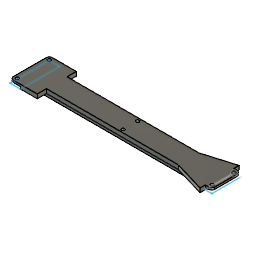
Carsen x10eb Mount1 (Autodesk Fusion 360 design; units mm, degrees)
part number: 2026-08-02-16-37-13-928
Autodesk Fusion 360 part; units mm, degrees
sketch "Skizze1" plane through (0, 0, 0) normal (0, 0, 1) x (1, 0, 0)
  line L0 (0, 27.8) -> (3.3, 27.8)
  line L1 (6.3, 24.8) -> (6.3, 3)
  line L2 (3.3, 0) -> (0, 0)
  line L3 (0, 0) -> (0, 27.8)
  circle A0 centre (3.3, 24.3) radius 1.575
  circle A1 centre (3.3, 3.5) radius 1.575
  line L4 (0, -5.025) -> (-180.6991, -5.025)
  line L5 (-183.6991, -2.025) -> (-183.6991, 29.825)
  line L6 (-180.6991, 32.825) -> (0, 32.825)
  line L7 (0, 32.825) -> (0, -5.025)
  circle A2 centre (-180.1991, 29.325) radius 1.575
  circle A3 centre (-180.1991, -1.525) radius 1.575
  arc A4 (6.3, 24.8) -> (3.3, 27.8) centre (3.3, 24.8) ccw
  arc A5 (3.3, 0) -> (6.3, 3) centre (3.3, 3) ccw
  arc A6 (-180.6991, 32.825) -> (-183.6991, 29.825) centre (-180.6991, 29.825) ccw
  arc A7 (-183.6991, -2.025) -> (-180.6991, -5.025) centre (-180.6991, -2.025) ccw
  line L8 (0, 23.9) -> (-183.6991, 23.9)
  line L9 (-183.6991, 23.9) -> (-183.6991, 3.9)
  line L10 (-183.6991, 3.9) -> (0, 3.9)
  line L11 (0, 3.9) -> (0, 23.9)
  line L12 (0, -5.025) -> (-30, 3.9)
  line L13 (0, 32.825) -> (-30, 23.9)
  line L14 (-30, 23.9) -> (-30, 32.825)
  line L15 (-30, -5.025) -> (-30, 3.9)
  line L16 (-157.4811, -5.025) -> (-157.4811, 3.9)
  line L17 (-157.4811, 23.9) -> (-157.4811, 32.825)
  dimension "d24" = 27.8
  dimension "d25" = 3.15
  dimension "d26" = 3.15
  dimension "d27" = 3.5
  dimension "d28" = 3.5
  dimension "d29" = 3
  dimension "d31" = 6.3
  dimension "d32" = 37.85
  dimension "d38" = 3.15
  dimension "d39" = 3.15
  dimension "d40" = 3.5
  dimension "d41" = 3.5
  dimension "d42" = 3.5
  dimension "d50" = 3
  dimension "d51" = 3
  dimension "d52" = 3
  dimension "d53" = 189.9991
  dimension "d54" = 8.925
  dimension "d55" = 8.925
  dimension "d56" = 30
  dimension "d57" = 30
  constraint horizontal L0
  constraint vertical L1
  constraint horizontal L2
  constraint vertical L3
  constraint vertical A0.centre A1.centre
  constraint horizontal L2.end L3.start
  constraint horizontal L4
  constraint vertical L5
  constraint horizontal L6
  constraint vertical L7
  constraint coincident L3 L4.start
  constraint midpoint L3 L7
  constraint vertical A2.centre A3.centre
  constraint tangent L0 A4
  constraint tangent L1 A4
  constraint tangent L1 A5
  constraint tangent L2 A5
  constraint tangent L6 A6
  constraint tangent L5 A6
  constraint tangent L5 A7
  constraint tangent L4 A7
  constraint equal A6 A7
  constraint vertical L2.end L4.start
  constraint horizontal L8
  constraint vertical L9
  constraint horizontal L10
  constraint vertical L11
  constraint coincident L5 L9.end
  constraint coincident L3 L8.start
  constraint coincident L10 L12.end
  constraint coincident L8 L13.end
  constraint coincident L6 L14.end
  constraint perpendicular L6 L14
  constraint perpendicular L4 L15
  constraint coincident L4 L15.start
  constraint coincident L4 L16.start
  constraint perpendicular L4 L16
  constraint coincident L10 L16.end
  constraint coincident L8 L17.start
  constraint perpendicular L8 L17
  constraint coincident L6 L17.end
  measures "d24" distance of L0 L2
  measures "d25" diameter of A0
  measures "d26" diameter of A1
  measures "d27" distance of L2 A1.centre
  measures "d28" distance of L0 A0.centre
  measures "d29" distance of L1 A0.centre
  measures "d31" distance of L1 L3
  measures "d32" distance of L4 L6
  measures "d38" diameter of A2
  measures "d39" diameter of A3
  measures "d40" distance of L6 A2.centre
  measures "d41" distance of L4 A3.centre
  measures "d42" distance of L5 A2.centre
  measures "d50" radius of A4
  measures "d51" radius of A5
  measures "d52" radius of A6
  measures "d53" distance of L1 L5
  measures "d54" distance of L4 L10
  measures "d55" distance of L6 L8
  measures "d56" horizontal distance of L4.start L12.end
  measures "d57" horizontal distance of L6.end L13.end
extrude "Extrusion8" add sketch "Skizze1" along normal blind 4 contours L0 L1 L2 L3 L7 A4 A5 L11 | L3 L7 L8 L13 | L3 L5 L7 L8 L9 L10 L11 | L3 L7 L10 L12 | L5 L6 A6 L8 L17 | L4 L5 A7 L10 L16
sketch "Skizze4" plane through (0, 0, 4) normal (0, 0, 1) x (-1, 0, 0)
  circle A0 centre (180.1991, 1.525) radius 1.575
  circle A1 centre (180.1991, -29.325) radius 1.575
  circle A2 centre (-3.3, -24.3) radius 1.575
  circle A3 centre (-3.3, -3.5) radius 1.575
  line L0 (0, -32.825) -> (30, -23.9)
  line L1 (30, -23.9) -> (157.4811, -23.9)
  line L2 (157.4811, -23.9) -> (157.4811, -32.825)
  line L3 (157.4811, -32.825) -> (180.6991, -32.825)
  arc A4 (180.6991, -32.825) -> (183.6991, -29.825) centre (180.6991, -29.825) ccw
  line L4 (183.6991, -29.825) -> (183.6991, -23.9)
  line L5 (183.6991, -23.9) -> (183.6991, -3.9)
  line L6 (183.6991, -3.9) -> (183.6991, 2.025)
  arc A5 (183.6991, 2.025) -> (180.6991, 5.025) centre (180.6991, 2.025) ccw
  line L7 (180.6991, 5.025) -> (157.4811, 5.025)
  line L8 (157.4811, 5.025) -> (157.4811, -3.9)
  line L9 (157.4811, -3.9) -> (30, -3.9)
  line L10 (30, -3.9) -> (0, 5.025)
  line L11 (0, 5.025) -> (0, 0)
  line L12 (0, 0) -> (-3.3, 0)
  arc A6 (-3.3, 0) -> (-6.3, -3) centre (-3.3, -3) ccw
  line L13 (-6.3, -3) -> (-6.3, -24.8)
  arc A7 (-6.3, -24.8) -> (-3.3, -27.8) centre (-3.3, -24.8) ccw
  line L14 (-3.3, -27.8) -> (0, -27.8)
  line L15 (0, -27.8) -> (0, -32.825)
  circle A8 centre (86.2, -6.9) radius 1.575
  circle A9 centre (86.2, -20.9) radius 1.575
  dimension "d60" = 3.15
  dimension "d61" = 92.5
  dimension "d63" = 3
  dimension "d64" = 3.15
  dimension "d65" = 92.5
  dimension "d66" = 3
  measures "d60" diameter of A8
  measures "d61" distance of L13 A8.centre
  measures "d63" distance of L9 A8.centre
  measures "d64" diameter of A9
  measures "d65" distance of L13 A9.centre
  measures "d66" distance of L1 A9.centre
extrude "Extrusion9" cut sketch "Skizze4" against normal blind 4 contours A8 | A9
sketch "Skizze5" plane through (0, 0, 0) normal (0, 0, -1) x (1, 0, 0)
  circle A0 centre (-86.2, -6.9) radius 1.575
  circle A1 centre (-86.2, -20.9) radius 1.575
  circle A2 centre (3.3, -3.5) radius 1.575
  circle A3 centre (-180.1991, -29.325) radius 1.575
  circle A4 centre (3.3, -24.3) radius 1.575
  circle A5 centre (-180.1991, 1.525) radius 1.575
  line L0 (-30, -23.9) -> (0, -32.825)
  line L1 (0, -32.825) -> (0, -27.8)
  line L2 (0, -27.8) -> (3.3, -27.8)
  arc A6 (3.3, -27.8) -> (6.3, -24.8) centre (3.3, -24.8) ccw
  line L3 (6.3, -24.8) -> (6.3, -3)
  arc A7 (6.3, -3) -> (3.3, 0) centre (3.3, -3) ccw
  line L4 (3.3, 0) -> (0, 0)
  line L5 (0, 0) -> (0, 5.025)
  line L6 (0, 5.025) -> (-30, -3.9)
  line L7 (-30, -3.9) -> (-157.4811, -3.9)
  line L8 (-157.4811, -3.9) -> (-157.4811, 5.025)
  line L9 (-157.4811, 5.025) -> (-180.6991, 5.025)
  arc A8 (-180.6991, 5.025) -> (-183.6991, 2.025) centre (-180.6991, 2.025) ccw
  line L10 (-183.6991, 2.025) -> (-183.6991, -3.9)
  line L11 (-183.6991, -3.9) -> (-183.6991, -23.9)
  line L12 (-183.6991, -23.9) -> (-183.6991, -29.825)
  arc A9 (-183.6991, -29.825) -> (-180.6991, -32.825) centre (-180.6991, -29.825) ccw
  line L13 (-180.6991, -32.825) -> (-157.4811, -32.825)
  line L14 (-157.4811, -32.825) -> (-157.4811, -23.9)
  line L15 (-157.4811, -23.9) -> (-30, -23.9)
  line L16 (0, -27.8) -> (6.5, -27.8)
  line L17 (6.5, -27.8) -> (6.5, 0)
  line L18 (6.5, 0) -> (0, 0)
  line L19 (0, 0) -> (0, -27.8)
  line L20 (-183.6991, -32.9017) -> (-173.6991, -32.9017)
  line L21 (-173.6991, -32.9017) -> (-173.6991, 5.078)
  line L22 (-173.6991, 5.078) -> (-183.6991, 5.078)
  line L23 (-183.6991, 5.078) -> (-183.6991, -32.9017)
  dimension "d69" = 10
  constraint horizontal L16
  constraint vertical L17
  constraint horizontal L18
  constraint vertical L19
  constraint coincident L1.end L2.start
  constraint horizontal L20
  constraint vertical L21
  constraint horizontal L22
  constraint vertical L23
  measures "d69" distance of L20.start L20.end
extrude "Extrusion10" cut sketch "Skizze5" against normal blind 2 contours L9 A8 L10 L11 L12 A9 L13 L21 L23
extrude "Extrusion11" cut sketch "Skizze5" against normal blind 2 contours L2 A6 L3 A7 L4 L16 L18 L19
sketch "Skizze6" plane through (0, 0, 0) normal (0, 0, -1) x (1, 0, 0)
  line L0 (-1.6975, -23.4) -> (-173.6975, -23.4)
  line L1 (-173.6975, -23.4) -> (-173.6975, -20.4)
  line L2 (-173.6975, -20.4) -> (-1.6975, -20.4)
  line L3 (-1.6975, -20.4) -> (-1.6975, -23.4)
  line L4 (0, 0) -> (0, -27.8)
  line L5 (-173.6991, -32.9017) -> (-173.6991, 5.078)
  line L6 (-157.4811, -23.9) -> (-30, -23.9)
  line L7 (-1.641, -4.4) -> (-173.641, -4.4)
  line L8 (-173.641, -4.4) -> (-173.641, -7.4)
  line L9 (-173.641, -7.4) -> (-1.641, -7.4)
  line L10 (-1.641, -7.4) -> (-1.641, -4.4)
  line L11 (-30, -3.9) -> (-157.4811, -3.9)
  line L12 (-73.2, -20.4) -> (-76.2, -20.4)
  line L13 (-76.2, -20.4) -> (-76.2, -7.4)
  line L14 (-76.2, -7.4) -> (-73.2, -7.4)
  line L15 (-73.2, -7.4) -> (-73.2, -20.4)
  line L16 (-33.3271, -20.4) -> (-73.2, -8.955)
  line L17 (-67.7437, -7.4) -> (-22.4534, -20.4)
  line L18 (-76.2, -20.4) -> (-96.2, -20.4)
  line L19 (-96.2, -20.4) -> (-96.2, -19)
  line L20 (-96.2, -19) -> (-76.2, -19)
  line L21 (-76.2, -19) -> (-76.2, -20.4)
  line L22 (-76.2, -7.4) -> (-96.2, -7.4)
  line L23 (-96.2, -7.4) -> (-96.2, -8.8)
  line L24 (-96.2, -8.8) -> (-76.2, -8.8)
  line L25 (-76.2, -8.8) -> (-76.2, -7.4)
  line L26 (-173.6975, -23.4) -> (-168.6975, -23.4)
  line L27 (-168.6975, -23.4) -> (-168.6975, -7.4)
  line L28 (-168.6975, -7.4) -> (-173.6975, -7.4)
  line L29 (-173.6975, -7.4) -> (-173.6975, -23.4)
  line L30 (-22.4534, -20.4) -> (-27.4534, -20.4)
  line L31 (-27.4534, -20.4) -> (-27.4534, -7.4)
  line L32 (-27.4534, -7.4) -> (-22.4534, -7.4)
  line L33 (-22.4534, -7.4) -> (-22.4534, -20.4)
  line L34 (-168.6975, -20.4) -> (-99.2, -8.9486)
  line L35 (-168.6975, -17.3595) -> (-108.2541, -7.4)
  line L36 (-96.2, -20.4) -> (-99.2, -20.4)
  line L37 (-99.2, -20.4) -> (-99.2, -7.4)
  line L38 (-99.2, -7.4) -> (-96.2, -7.4)
  line L39 (-96.2, -7.4) -> (-96.2, -20.4)
  point P0 (-86.2, -20.9)
  dimension "d74" = 172
  dimension "d75" = 3
  dimension "d76" = 173.6991
  dimension "d78" = 0.5
  dimension "d81" = 3
  dimension "d82" = 0.5
  dimension "d83" = 3
  dimension "d85" = 10
  dimension "d88" = 3
  dimension "d90" = 20
  dimension "d91" = 1.4
  dimension "d92" = 5
  dimension "d93" = 172
  dimension "d96" = 3
  dimension "d101" = 5
  dimension "d102" = 13
  constraint horizontal L0
  constraint vertical L1
  constraint horizontal L2
  constraint vertical L3
  constraint horizontal L7
  constraint vertical L8
  constraint horizontal L9
  constraint vertical L10
  constraint horizontal L12
  constraint vertical L13
  constraint horizontal L14
  constraint vertical L15
  constraint coincident L2 L12.start
  constraint coincident L2 L16.start
  constraint coincident L15 L16.end
  constraint coincident L9 L17.start
  constraint coincident L2 L17.end
  constraint parallel L16 L17
  constraint horizontal L18
  constraint vertical L19
  constraint horizontal L20
  constraint vertical L21
  constraint horizontal L22
  constraint vertical L23
  constraint horizontal L24
  constraint vertical L25
  constraint horizontal L26
  constraint vertical L27
  constraint horizontal L28
  constraint vertical L29
  constraint horizontal L30
  constraint vertical L31
  constraint horizontal L32
  constraint vertical L33
  constraint coincident L9 L31.end
  constraint coincident L27 L34.start
  constraint coincident L2 L34.start
  constraint coincident L27 L35.start
  constraint coincident L9 L35.end
  constraint parallel L34 L35
  constraint horizontal L36
  constraint vertical L37
  constraint horizontal L38
  constraint vertical L39
  constraint coincident L9 L37.end
  measures "d74" distance of L0.start L0.end
  measures "d75" distance of L0.start L2.end
  measures "d76" distance of L4 L5
  measures "d78" distance of L0 L6
  measures "d81" distance of L7.start L9.end
  measures "d82" distance of L7 L11
  measures "d83" distance of L12.start L12.end
  measures "d85" distance of L13 P0
  measures "d88" distance of L16 L17
  measures "d90" distance of L13.end L22.end
  measures "d91" distance of L13.end L24.end
  measures "d92" distance of L0.end L26.end
  measures "d93" distance of L7.start L7.end
  measures "d96" distance of L34 L35
  measures "d101" distance of L31 L33
  measures "d102" distance of L2 L9
extrude "Extrusion12" add sketch "Skizze6" along normal blind 3 contours L0 L2 L3 L12 L18 L27 L30 L36 | L0 L1 L2 L5 L26 L27 L29
sketch "Skizze7" plane through (0, 0, 0) normal (0, 0, -1) x (1, 0, 0)
extrude "Extrusion15" add sketch "Skizze6" along normal blind 3 contours L2 L5 L9 L27 L28 L29 | L9 L27 L34 L35 L37 | L2 L17 L30 L31 | L9 L17 L31 L32 L33 | L2 L9 L19 L23 L36 L37 L38 L39 | L2 L9 L15 L16 L17 L31 | L7 L8 L9 L10 L14 L22 L28 L32 L38 | L2 L13 L18 L19 L20 L21 L39 | L2 L9 L12 L13 L14 L15 L21 L25 | L9 L13 L22 L23 L24 L25 L39
extrude "Extrusion16" cut sketch "Skizze5" along normal blind 4 contours A0 | A1
extrude "Extrusion13" [suppressed]
extrude "Extrusion14" [suppressed]
extrude "Extrusion4" [suppressed]
extrude "Extrusion5" [suppressed]
extrude "Extrusion1" [suppressed]
extrude "Extrusion2" [suppressed]
extrude "Extrusion3" [suppressed]
sketch "Skizze3" plane through (0, 0, 0) normal (0, 0, 1) x (1, 0, 0)
equation "d27 = 2 mm + 1.5 mm"
